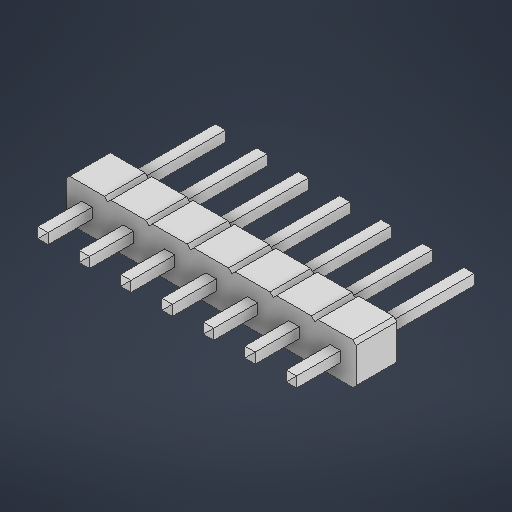
# Autodesk Inventor part: Barra de pinos
Saved by Autodesk Inventor 2027 (Build 310192000, 192)
## iProperties
Created: 2026-06-25
Part Number: Barra de pinos
Material: Genérico
Document SubType Name: Modeling
Designer: marcu
Density: 1 g/cm^3
Appearance: Padrão
Author: marcu
Autodesk Inventor part; units mm, degrees
ref_plane "YZ Plane" through (0, 0, 0) normal (1, 0, 0) x (0, 1, 0)
ref_plane "XZ Plane" through (0, 0, 0) normal (0, 1, 0) x (-1, 0, 0)
ref_plane "XY Plane" through (0, 0, 0) normal (0, 0, 1) x (1, 0, 0)
sketch "Esboço4" plane through (0, 0, 0) normal (0, 0, 1) x (1, 0, 0)
  line L0 (-1.27, 1.27) -> (1.27, 1.27)
  line L1 (1.27, 1.27) -> (1.27, -1.27)
  line L2 (1.27, -1.27) -> (-1.27, -1.27)
  line L3 (-1.27, -1.27) -> (-1.27, 1.27)
  line L4 (-1.27, 1.27) -> (1.27, -1.27) construction
  line L5 (1.27, 1.27) -> (-1.27, -1.27) construction
  point P0 (0, 0)
  dimension "d28" = 2.54
  dimension "d29" = 2.54
  constraints: 12 end point, 2 midpoint, 2 parallel, 1 horizontal, 1 perpendicular
  measures "d28" distance of L1.end L0.end
  measures "d29" distance of L0.end L0.start
extrude "Extrusão4" add sketch "Esboço4" along normal mid plane 2.5
chamfer "Chanfro5" distance 0.2 angle 45 4 edges at (-1.27, 1.27, 0) (-1.27, -1.27, 0) (1.27, 1.27, 0) (1.27, -1.27, 0)
sketch "Esboço7" plane through (0, 0, 1.25) normal (0, 0, 1) x (1, 0, 0)
  line L0 (0.32, 0.32) -> (-0.32, 0.32)
  line L1 (-0.32, 0.32) -> (-0.32, -0.32)
  line L2 (-0.32, -0.32) -> (0.32, -0.32)
  line L3 (0.32, -0.32) -> (0.32, 0.32)
  line L4 (0.32, 0.32) -> (-0.32, -0.32) construction
  line L5 (-0.32, 0.32) -> (0.32, -0.32) construction
  point P0 (0, 0)
  dimension "d41" = 0.64
  dimension "d42" = 0.64
  constraints: 12 end point, 2 midpoint, 2 parallel, 1 horizontal, 1 perpendicular
  measures "d41" distance of L2.end L0.start
  measures "d42" distance of L0.end L0.start
extrude "Extrusão7" add sketch "Esboço7" along normal blind 3
sketch "Esboço8" plane through (0, 0, -1.25) normal (0, 0, -1) x (-1, 0, 0)
  line L0 (-0.32, -0.32) -> (0.32, -0.32)
  line L1 (0.32, -0.32) -> (0.32, 0.32)
  line L2 (0.32, 0.32) -> (-0.32, 0.32)
  line L3 (-0.32, 0.32) -> (-0.32, -0.32)
  line L4 (-0.32, -0.32) -> (0.32, 0.32) construction
  line L5 (0.32, -0.32) -> (-0.32, 0.32) construction
  point P0 (0, 0)
  dimension "d45" = 0.64
  dimension "d46" = 0.64
  constraints: 12 end point, 2 midpoint, 2 parallel, 1 horizontal, 1 perpendicular
  measures "d45" distance of L2.end L0.start
  measures "d46" distance of L1.end L2.end
extrude "Extrusão8" add sketch "Esboço8" along normal blind 6
chamfer "Chanfro6" distance 0.3 angle 45 4 edges at (-0.32, 0, -7.25) (0, -0.32, -7.25) (0.32, 0, -7.25) (0, 0.32, -7.25)
chamfer "Chanfro7" distance 0.3 angle 45 4 edges at (0.32, 0, 4.25) (0, 0.32, 4.25) (-0.32, 0, 4.25) (0, -0.32, 4.25)
pattern_linear "Padrão retangular1" count 2 spacing 2.54 along (1, 0, 0) of "Extrusão8", "Extrusão4", "Extrusão7"
chamfer "Chanfro8" distance 0.3 angle 45 8 edges at (2.54, -0.32, -7.25) (2.86, 0, -7.25) (2.54, 0.32, -7.25) (2.22, 0, -7.25) (2.54, -0.32, 4.25) (2.86, 0, 4.25) (2.54, 0.32, 4.25) (2.22, 0, 4.25)
chamfer "Chanfro9" distance 0.2 angle 45 4 edges at (1.27, -1.27, 0) (3.81, -1.27, 0) (1.27, 1.27, 0) (3.81, 1.27, 0)
pattern_linear "Padrão retangular2" count 2 spacing 5.08 along (1, 0, 0) of "Extrusão7", "Extrusão8", "Extrusão4"
chamfer "Chanfro10" distance 0.2 angle 45 4 edges at (6.35, 1.27, 0) (3.81, 1.27, 0) (3.81, -1.27, 0) (6.35, -1.27, 0)
chamfer "Chanfro11" distance 0.3 angle 45 8 edges at (5.08, -0.32, 4.25) (5.4, 0, 4.25) (5.08, 0.32, 4.25) (4.76, 0, 4.25) (4.76, 0, -7.25) (5.08, 0.32, -7.25) (5.4, 0, -7.25) (5.08, -0.32, -7.25)
pattern_linear "Padrão retangular3" count 2 spacing 7.62 along (1, 0, 0) of "Extrusão7", "Extrusão8", "Extrusão4"
chamfer "Chanfro12" distance 0.3 angle 45 8 edges at (7.62, 0.32, -7.25) (7.3, 0, -7.25) (7.62, -0.32, -7.25) (7.94, 0, -7.25) (7.62, -0.32, 4.25) (7.94, 0, 4.25) (7.62, 0.32, 4.25) (7.3, 0, 4.25)
chamfer "Chanfro13" distance 0.2 angle 45 4 edges at (6.35, -1.27, 0) (8.89, -1.27, 0) (6.35, 1.27, 0) (8.89, 1.27, 0)
pattern_linear "Padrão retangular4" count 2 spacing 10.16 along (1, 0, 0) of "Extrusão7", "Extrusão8", "Extrusão4"
chamfer "Chanfro14" distance 0.2 angle 45 4 edges at (8.89, 1.27, 0) (11.43, 1.27, 0) (8.89, -1.27, 0) (11.43, -1.27, 0)
chamfer "Chanfro15" distance 0.3 angle 45 8 edges at (10.16, -0.32, 4.25) (10.48, 0, 4.25) (10.16, 0.32, 4.25) (9.84, 0, 4.25) (10.16, 0.32, -7.25) (10.48, 0, -7.25) (10.16, -0.32, -7.25) (9.84, 0, -7.25)
pattern_linear "Padrão retangular5" count 2 spacing 12.7 along (1, 0, 0) of "Extrusão8", "Extrusão7", "Extrusão4"
chamfer "Chanfro16" distance 0.3 angle 45 8 edges at (12.7, -0.32, -7.25) (12.38, 0, -7.25) (12.7, 0.32, -7.25) (13.02, 0, -7.25) (12.38, 0, 4.25) (12.7, 0.32, 4.25) (13.02, 0, 4.25) (12.7, -0.32, 4.25)
chamfer "Chanfro17" distance 0.2 angle 45 4 edges at (11.43, -1.27, 0) (13.97, -1.27, 0) (11.43, 1.27, 0) (13.97, 1.27, 0)
pattern_linear "Padrão retangular6" count 2 spacing 15.24 along (1, 0, 0) of "Extrusão8", "Extrusão7", "Extrusão4"
chamfer "Chanfro18" distance 0.2 angle 45 4 edges at (13.97, -1.27, 0) (16.51, -1.27, 0) (13.97, 1.27, 0) (16.51, 1.27, 0)
chamfer "Chanfro19" distance 0.3 angle 45 8 edges at (15.24, 0.32, -7.25) (15.56, 0, -7.25) (15.24, -0.32, -7.25) (14.92, 0, -7.25) (15.24, -0.32, 4.25) (15.56, 0, 4.25) (15.24, 0.32, 4.25) (14.92, 0, 4.25)
